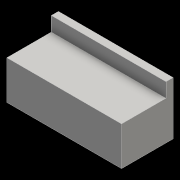
# Autodesk Inventor part: cushion
Saved by Autodesk Inventor 2016 (Build 200138000, 138)
## iProperties
Created: 2019-02-12
Part Number: cushion
Material: Generic
Document SubType Name: Modeling
Designer: Calb3e
Density: 1 g/cm^3
Appearance: Default
Author: Calb3e
Autodesk Inventor part; units mm, degrees
ref_plane "YZ Plane" through (0, 0, 0) normal (1, 0, 0) x (0, 1, 0)
ref_plane "XZ Plane" through (0, 0, 0) normal (0, 1, 0) x (-1, 0, 0)
ref_plane "XY Plane" through (0, 0, 0) normal (0, 0, 1) x (1, 0, 0)
sketch "Sketch1" plane through (0, 0, 0) normal (0, 1, 0) x (-1, 0, 0)
  line L0 (0, 0) -> (-80, 0)
  line L1 (-80, 0) -> (-80, -37)
  line L2 (-80, -37) -> (0, -37)
  line L3 (0, -37) -> (0, 0)
  dimension "d0" = 80
  dimension "d1" = 37
  constraints: 8 end point, 2 parallel, 1 horizontal, 1 perpendicular
  measures "d0" distance of L2.end L1.end
  measures "d1" distance of L1.end L0.end
extrude "Extrusion1" add sketch "Sketch1" along normal blind 36
sketch "Sketch2" plane through (80, 0, 0) normal (1, 0, 0) x (0, 0, -1)
  line L0 (0, 0) -> (37, 0) projected
  line L1 (37, 0) -> (37, 36) projected
  line L2 (0, 36) -> (37, 36) projected
  line L3 (0, 0) -> (0, 36) projected
  line L4 (0, 0) -> (10, 0)
  line L5 (10, 0) -> (10, 31)
  line L6 (10, 31) -> (0, 31)
  line L7 (0, 31) -> (0, 0)
  dimension "d4" = 5
  dimension "d5" = 27
  constraints: 8 end point, 2 parallel, 1 horizontal, 1 perpendicular
  measures "d4" distance between parallel lines of L6 L2
  measures "d5" distance between parallel lines of L1 L5
extrude "Extrusion2" cut sketch "Sketch2" against normal through all contours L3 L6 L5 L0
body "Solid1"
